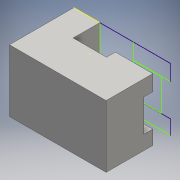
# Autodesk Inventor part: 240503_3Dsketch06
Saved by Autodesk Inventor 2016 (Build 200138000, 138)
## iProperties
Created: 2024-05-03
Part Number: 240503_3Dsketch06
Material: 일반
Document SubType Name: Modeling
Designer: pc
Density: 1 g/cm^3
Appearance: 기본값
Author: pc
Autodesk Inventor part; units mm, degrees
ref_plane "YZ Plane" through (0, 0, 0) normal (1, 0, 0) x (0, 1, 0)
ref_plane "XZ Plane" through (0, 0, 0) normal (0, 1, 0) x (-1, 0, 0)
ref_plane "XY Plane" through (0, 0, 0) normal (0, 0, 1) x (1, 0, 0)
sketch "스케치1" plane through (0, 0, 0) normal (0, 0, 1) x (1, 0, 0)
  line L0 (54.3328, -36.1894) -> (-54.3328, -36.1894)
  line L1 (-54.3328, -36.1894) -> (-54.3328, 36.1894)
  line L2 (-54.3328, 36.1894) -> (54.3328, 36.1894)
  line L3 (54.3328, 36.1894) -> (54.3328, -36.1894)
  line L4 (54.3328, -36.1894) -> (-54.3328, 36.1894) construction
  line L5 (-54.3328, -36.1894) -> (54.3328, 36.1894) construction
  point P0 (0, 0)
  constraints: 12 end point, 2 midpoint, 2 parallel, 1 horizontal, 1 perpendicular
extrude "돌출1" add sketch "스케치1" along normal blind 70
sketch "스케치2" plane through (-54.3328, 36.1894, 0) normal (0, 1, 0) x (1, 0, 0)
  line L0 (0, -70) -> (108.6655, -70) projected
  line L1 (108.6655, 0) -> (0, 0) projected
  line L2 (29.224, -70) -> (66.7649, -70)
  line L3 (66.7649, -70) -> (66.7649, 0)
  line L4 (66.7649, 0) -> (29.224, 0)
  line L5 (29.224, 0) -> (29.224, -70)
  line L6 (66.7649, -52.0222) -> (98.3413, -52.0222)
  line L7 (98.3413, -52.0222) -> (98.3413, -16.2356)
  line L8 (98.3413, -16.2356) -> (66.7649, -16.2356)
  line L9 (66.7649, -16.2356) -> (66.7649, -52.0222)
  point P0 (54.3328, 0)
  constraints: 16 end point, 4 parallel, 3 point on line, 2 horizontal, 2 perpendicular
extrude "돌출2" cut sketch "스케치2" against normal blind 30 contours L5 L1 L3 L0
sketch "스케치3" plane through (54.3328, 36.1894, 70) normal (0, 1, 0) x (1, 0, 0)
  line L0 (-41.9007, 70) -> (-41.9007, 0) projected
  line L1 (0, 70) -> (0, 0) projected
  line L2 (-41.9007, 53.9806) -> (0, 53.9806)
  line L3 (0, 53.9806) -> (0, 17.7133)
  line L4 (0, 17.7133) -> (-41.9007, 17.7133)
  line L5 (-41.9007, 17.7133) -> (-41.9007, 53.9806)
  point P0 (-54.3328, 70)
  constraints: 8 end point, 2 parallel, 2 point on line, 1 horizontal, 1 perpendicular
extrude "돌출3" cut sketch "스케치3" against normal blind 30
sketch "스케치4" plane through (0, 0, 70) normal (0, 0, 1) x (1, 0, 0)
  point P0 (0, 0)
sketch "스케치5" plane through (12.4321, 36.1894, 0) normal (0, 1, 0) x (1, 0, 0)
  line L0 (41.9007, 0) -> (41.9007, -16.0194) projected
  line L1 (0, 0) -> (41.9007, 0)
  line L2 (41.9007, 0) -> (41.9007, -16.0194)
  line L3 (41.9007, -16.0194) -> (0, -16.0194)
  line L4 (0, -16.0194) -> (0, 0)
  line L5 (41.9007, -70) -> (0, -70) projected
  line L6 (0, -52.2867) -> (41.9007, -52.2867)
  line L7 (41.9007, -52.2867) -> (41.9007, -70)
  line L8 (41.9007, -70) -> (0, -70)
  line L9 (0, -70) -> (0, -52.2867)
  point P0 (-12.4321, 0)
  constraints: 16 end point, 4 parallel, 2 horizontal, 2 perpendicular, 1 point on line
extrude "돌출4" cut sketch "스케치5" against normal blind 20 contours L0 L3 L4 L1
extrude "돌출5" cut sketch "스케치5" against normal blind 20 contours L5 L9 L6 L7
